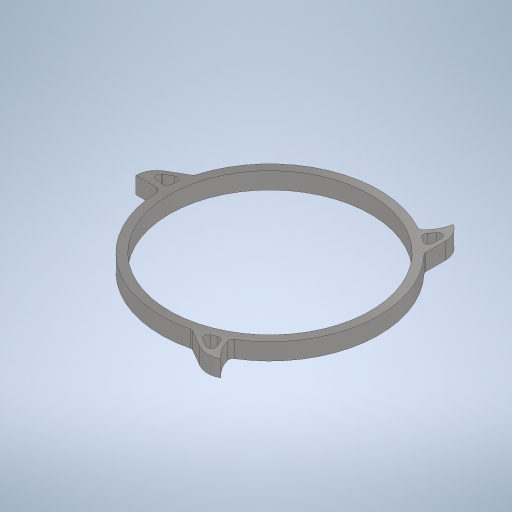
# Autodesk Inventor part: Ring
Saved by Autodesk Inventor 2023.2 (Build 272271000, 271)
## iProperties
Created: 2023-04-12
Part Number: Ring
Material: Stainless Steel
Document SubType Name: Modeling
Designer: Nathan Cai
Mass: 375.749 g
Surface Area: 225.589 cm^2
Volume: 46.9686 cm^3
Density: 8 g/cm^3
Appearance: Semi-Polished
Author: Nathan Cai
Autodesk Inventor part; units mm, degrees
ref_plane "YZ Plane" through (0, 0, 0) normal (1, 0, 0) x (0, 1, 0)
ref_plane "XZ Plane" through (0, 0, 0) normal (0, 1, 0) x (-1, 0, 0)
ref_plane "XY Plane" through (0, 0, 0) normal (0, 0, 1) x (1, 0, 0)
sketch "Sketch1" plane through (0, 0, 0) normal (0, 1, 0) x (-1, 0, 0)
  circle A0 centre (0, 0) radius 76.2
  circle A1 centre (0, 0) radius 82.55
  line L0 (0, 0) -> (101.6, 0)
  arc A2 (82.55, 0) -> (101.6, 0) centre (92.075, 26.1697) ccw
  line L1 (101.6, 0) -> (92.4836, -3.3181) construction
  arc A3 (93.6625, -13.7482) -> (101.6, 0) centre (85.725, 0) ccw
  line L2 (93.6625, -13.7482) -> (79.6013, -21.8664)
  arc A4 (92.075, -10.9985) -> (98.3891, -0.9543) centre (85.725, 0) ccw
  line L3 (92.075, -10.9985) -> (80.6536, -17.5927)
  arc A5 (82.4826, -3.3343) -> (101.2144, -3.4778) centre (92.075, 26.1697) ccw
  arc A6 (-41.275, 71.4904) -> (-50.8, 87.9882) centre (-68.7011, 66.6544) ccw
  line L4 (-50.8, 87.9882) -> (-43.3683, 81.7522) construction
  arc A7 (-34.925, 87.9882) -> (-50.8, 87.9882) centre (-42.8625, 74.24) ccw
  line L5 (-34.925, 87.9882) -> (-20.8638, 79.8699)
  arc A8 (-36.5125, 85.2386) -> (-48.3681, 85.6846) centre (-42.8625, 74.24) ccw
  line L6 (-36.5125, 85.2386) -> (-25.0911, 78.6444)
  arc A9 (-38.3537, 73.0992) -> (-47.5953, 89.3931) centre (-68.7011, 66.6544) ccw
  arc A10 (-41.275, -71.4904) -> (-50.8, -87.9882) centre (-23.3739, -92.8242) ccw
  line L7 (-50.8, -87.9882) -> (-49.1154, -78.4341) construction
  arc A11 (-58.7375, -74.24) -> (-50.8, -87.9882) centre (-42.8625, -74.24) ccw
  line L8 (-58.7375, -74.24) -> (-58.7375, -58.0035)
  arc A12 (-55.5625, -74.24) -> (-50.021, -84.7303) centre (-42.8625, -74.24) ccw
  line L9 (-55.5625, -74.24) -> (-55.5625, -61.0517)
  arc A13 (-44.1289, -69.7649) -> (-53.619, -85.9153) centre (-23.3739, -92.8242) ccw
  point P0 (-20.8638, 79.8699)
  point P1 (-41.275, 71.4904)
  point P2 (-58.7375, -58.0035)
  point P3 (-41.275, -71.4904)
  point P4 (-44.1289, -69.7649)
  point P5 (-52.5943, -82.3998)
  point P6 (-55.5625, -61.0517)
  point P7 (-38.3537, 73.0992)
  point P8 (-45.0631, 86.7479)
  point P9 (-25.0911, 78.6444)
  point P10 (97.6575, -4.3481)
  dimension "d0" = 152.4
  dimension "d1" = 6.35
  dimension "d2" = 101.6
  dimension "d3" = 20
  dimension "d4" = 15.875
  dimension "d5" = 30
  dimension "d10" = 3.175
  dimension "d11" = 3.175
  dimension "d14" = 360
  constraints: 34 point on circle, 20 end point, 14 centre point, 3 tangent, 1 coincident, 1 horizontal, 1 line through centre, 1 parallel, 1 point on line, 58 other
  measures "d0" diameter of A0
  measures "d1" radial gap between concentric circles of A0 A1
  measures "d2" distance of L0.start L0.end
  measures "d3" angle of L0 L1
  measures "d4" radius of A3
  measures "d5" angle of L0 L2
  measures "d10" radial gap between concentric circles of A3 A4
  measures "d11" radial gap between concentric circles of A2 A5
extrude "Extrusion1" add sketch "Sketch1" along normal blind 12.7 contours A1 | A2 A4 A5 A1 | L0 A2 | A1 L6 A8 A9 A7 L5 | A3 A5 A4 A2 | L3 A4 A5 A3 L2 A1 | A1 A6 A8 A9 | A9 A8 A6 A7 | A10 A12 A13 A1 | A1 L9 A12 A13 A11 L8 | A10 A11 A13 A12
fillet "Fillet1" radius 3.175 15 edges at (41.275, 6.35, 71.4904) (38.3537, 6.35, 73.0992) (25.0911, 6.35, 78.6444) (45.0631, 6.35, 86.7479) (52.5943, 6.35, -82.3998) (55.5625, 6.35, -61.0517) (44.1289, 6.35, -69.7649) (41.275, 6.35, -71.4904) (-79.6013, 6.35, -21.8664) (-80.6536, 6.35, -17.5927) (-82.4826, 6.35, -3.3343) (-97.6575, 6.35, -4.3481) (-82.55, 6.35, 0) (58.7375, 6.35, -58.0035) (20.8638, 6.35, 79.8699)
equation "\"d10\" = d11"
body "Solid1"
